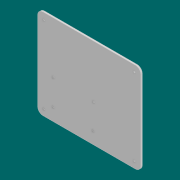
# Autodesk Inventor part: Back
Saved by Autodesk Inventor 2020.1 (Build 241239000, 239)
## iProperties
Created: 2019-07-23
Part Number: Back
Material: Generic
Document SubType Name: Modeling
Designer: Pluscrafter
Density: 1 g/cm^3
Appearance: Default
Author: Pluscrafter
Autodesk Inventor part; units mm, degrees
ref_plane "YZ Plane" through (0, 0, 0) normal (1, 0, 0) x (0, 1, 0)
ref_plane "XZ Plane" through (0, 0, 0) normal (0, 1, 0) x (-1, 0, 0)
ref_plane "XY Plane" through (0, 0, 0) normal (0, 0, 1) x (1, 0, 0)
sketch "Sketch1" plane through (0, 0, 0) normal (0, 0, 1) x (1, 0, 0)
  line L0 (-6.4664, 150.0295) -> (163.5336, 150.0295) construction
  line L1 (173.5336, 140.0295) -> (173.5336, -4.9705) construction
  line L2 (163.5336, -14.9705) -> (-6.4664, -14.9705)
  line L3 (-16.4664, -4.9705) -> (-16.4664, 140.0295)
  arc A0 (-6.4664, 150.0295) -> (-16.4664, 140.0295) centre (-6.4664, 140.0295) ccw
  arc A1 (173.5336, 140.0295) -> (163.5336, 150.0295) centre (163.5336, 140.0295) ccw construction
  arc A2 (163.5336, -14.9705) -> (173.5336, -4.9705) centre (163.5336, -4.9705) ccw
  arc A3 (-16.4664, -4.9705) -> (-6.4664, -14.9705) centre (-6.4664, -4.9705) ccw
  line L4 (-16.4664, 140.0295) -> (173.5336, 140.0295) construction
  line L5 (-16.4664, -4.9705) -> (173.5336, -4.9705) construction
  line L6 (-6.4664, -14.9705) -> (-6.4664, 150.0295) construction
  line L7 (163.5336, 150.0295) -> (163.5336, -14.9705) construction
  circle A4 centre (-6.4664, 140.0295) radius 1.5
  circle A5 centre (163.5336, 140.0295) radius 1.5
  circle A6 centre (163.5336, -4.9705) radius 1.5
  circle A7 centre (-6.4664, -4.9705) radius 1.5
  circle A8 centre (11.0336, 7.0295) radius 1.5
  circle A9 centre (86.0336, 5.7795) radius 1.5
  circle A10 centre (11.0336, 55.2351) radius 1.5
  circle A11 centre (87.0336, 52.9745) radius 1.5
  line L8 (-8.4664, -16.9705) -> (165.5336, -16.9705)
  line L9 (175.5336, -6.9705) -> (175.5336, 142.0295)
  line L10 (165.5336, 152.0295) -> (-8.4664, 152.0295)
  line L11 (-18.4664, 142.0295) -> (-18.4664, -6.9705)
  arc A12 (-8.4664, 152.0295) -> (-18.4664, 142.0295) centre (-8.4664, 142.0295) ccw
  arc A13 (-18.4664, -6.9705) -> (-8.4664, -16.9705) centre (-8.4664, -6.9705) ccw
  arc A14 (165.5336, -16.9705) -> (175.5336, -6.9705) centre (165.5336, -6.9705) ccw
  arc A15 (175.5336, 142.0295) -> (165.5336, 152.0295) centre (165.5336, 142.0295) ccw
  point P0 (0, 0)
  point P1 (173.5336, -14.9705)
  point P2 (173.5336, 150.0295)
  point P3 (-16.4664, -14.9705)
  point P4 (-18.4664, -16.9705)
  point P5 (175.5336, 152.0295)
  point P6 (-18.4664, 152.0295)
  dimension "d0" = 190
  dimension "d1" = 165
  dimension "d2" = 10
  dimension "a" = 3
  dimension "d4" = 3
  dimension "d5" = 3
  dimension "d6" = 3
  dimension "d7" = 3
  dimension "d8" = 3
  dimension "d9" = 3
  dimension "d10" = 3
  dimension "d11" = 12
  dimension "d12" = 10.75
  dimension "d14" = 75
  dimension "d16" = 76
  dimension "d17" = 194
  dimension "d18" = 169
  dimension "d19" = 2
  dimension "d20" = 2
  dimension "d21" = 10
  dimension "d24" = 29.5
  dimension "d25" = 29.5
  constraints: 24 end point, 17 point on circle, 16 centre point, 16 tangent, 12 point on line, 6 equal radius, 6 parallel, 4 coincident, 3 horizontal, 2 perpendicular
  measures "d0" distance of point (173.534, -14.971) point (-16.466, -14.971)
  measures "d1" distance of point (173.534, 150.029) point (173.534, -14.971)
  measures "d2" radius of A0
  measures "a" diameter of A4
  measures "d4" diameter of A5
  measures "d5" diameter of A6
  measures "d6" diameter of A7
  measures "d7" diameter of A8
  measures "d8" diameter of A9
  measures "d9" diameter of A10
  measures "d10" diameter of A11
  measures "d11" distance from line of A8.centre L5
  measures "d12" distance from line of L5 A9.centre
  measures "d14" horizontal distance of A9.centre A8.centre
  measures "d16" horizontal distance of A11.centre A10.centre
  measures "d17" distance of point (-18.466, 152.029) point (175.534, 152.029)
  measures "d18" distance of point (-18.466, 152.029) point (-18.466, -16.971)
  measures "d19" distance between parallel lines of L3 L11
  measures "d20" distance between parallel lines of L0 L10
  measures "d21" radius of A12
  measures "d24" distance from line of L11 A10.centre
  measures "d25" distance from line of L11 A8.centre
extrude "Extrusion1" add sketch "Sketch1" along normal blind 3
equation "\"d4\" = a"
equation "\"d5\" = a"
equation "\"d6\" = a"
equation "\"d7\" = a"
equation "\"d8\" = a"
equation "\"d9\" = a"
equation "\"d10\" = a"
body "Solid1"
